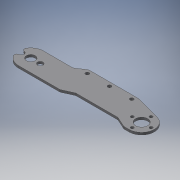
# Autodesk Inventor part: rinnku
Saved by Autodesk Inventor 2018 (Build 220112000, 112)
## iProperties
Created: 2016-08-23
Part Number: rinnku
Material: GFRP
Document SubType Name: Modeling
Designer: hiro
Density: 1.75 g/cm^3
Appearance: 滑らか - 淡い灰色
Mass: 9.22094 g
Surface Area: 59.6576 cm^2
Volume: 5.26911 cm^3
Author: hiro
Autodesk Inventor part; units mm, degrees
ref_plane "YZ Plane" through (0, 0, 0) normal (1, 0, 0) x (0, 1, 0)
ref_plane "XZ Plane" through (0, 0, 0) normal (0, 1, 0) x (-1, 0, 0)
ref_plane "XY Plane" through (0, 0, 0) normal (0, 0, 1) x (1, 0, 0)
sketch "スケッチ1" plane through (0, 0, 0) normal (0, 0, 1) x (1, 0, 0)
  line L0 (-50, 0) -> (50, 0) construction
  circle A0 centre (-50, 0) radius 4
  circle A1 centre (50, 0) radius 5.55
  line L1 (-50, 11.35) -> (-23, 11.35)
  line L2 (-50, -11.35) -> (50, -11.35)
  arc A2 (50, -11.35) -> (50, 11.35) centre (50, 0) ccw
  line L3 (30, 17) -> (-15, 17)
  line L4 (-15, 17) -> (-23, 11.35)
  line L5 (-24.9115, 10) -> (41.8474, 10) construction
  line L6 (-15, 17) -> (-15, 10) construction
  line L7 (30, 17) -> (30, 10) construction
  circle A3 centre (27.5, 13.5) radius 1.55
  circle A4 centre (-12.5, 13.5) radius 1.55
  circle A5 centre (7.5, 13.5) radius 1.55
  line L8 (-15, 13.5) -> (30, 13.5) construction
  line L9 (30, 16) -> (-15, 16) construction
  line L10 (-15, 16) -> (-15, 11) construction
  line L11 (-15, 11) -> (30, 11) construction
  line L12 (30, 11) -> (30, 16) construction
  line L13 (-23, 11.35) -> (50, 11.35)
  arc A6 (-50, 11.35) -> (-50, -11.35) centre (-50, 0) ccw
  line L14 (7.5, 17) -> (7.5, 10.5172) construction
  line L15 (30, 17) -> (52.8887, 10.9762)
  point P0 (0, 0)
  point P1 (0, 0)
  point P2 (55.7736, 9.7718)
  point P3 (38, 11.35)
  dimension "d0" = 100
  dimension "d1" = 8
  dimension "d8" = 11.1
  dimension "d10" = 7
  dimension "d11" = 45
  dimension "d12" = 2.5
  dimension "d13" = 3.1
  dimension "d14" = 2.5
  dimension "d15" = 20
  dimension "d17" = 5
  dimension "d18" = 11
  dimension "d69" = 11.35
  dimension "d72" = 11.35
  dimension "d87" = 8
  dimension "d88" = 8
  constraints: 32 end point, 8 point on line, 7 centre point, 7 horizontal, 6 midpoint, 6 point on circle, 5 coincident, 4 perpendicular, 4 tangent, 2 equal radius, 2 parallel
  measures "d0" distance of L0.start L0.end
  measures "d1" diameter of A0
  measures "d8" diameter of A1
  measures "d10" distance between parallel lines of L3 L5
  measures "d11" distance between parallel lines of L7 L6
  measures "d12" distance from line of A4.centre L6
  measures "d13" diameter of A4
  measures "d14" distance from line of L7 A3.centre
  measures "d15" distance from line of L7 L0.end
  measures "d17" distance between parallel lines of L9 L11
  measures "d18" distance between parallel lines of L0 L11
  measures "d69" radius of A2
  measures "d72" radius of A6
  measures "d87" horizontal distance of L3.start point (38, 11.35)
  measures "d88" horizontal distance of L3.end L1.end
extrude "押し出し1" add sketch "スケッチ1" along normal blind 2
fillet "フィレット1" radius 5 3 edges at (-23, 11.35, 1) (-15, 17, 1) (30, 17, 1)
sketch "スケッチ2" plane through (0, 0, 2) normal (0, 0, 1) x (1, 0, 0)
  arc A0 (50, -11.35) -> (52.8887, 10.9762) centre (50, 0) ccw projected
  line L0 (18, -20) -> (-35.4549, -20) construction
  line L1 (-76.9372, -11.5) -> (-72, -11.5)
  line L2 (-76.9372, -12.4) -> (-76.9372, -11.5)
  line L3 (-71.9872, -11.45) -> (-76.9872, -11.45)
  line L4 (-76.9872, -11.45) -> (-76.9872, -12.45)
  circle A1 centre (-50, 0) radius 4 projected
  circle A2 centre (-50, 0) radius 5.5 construction
  circle A3 centre (50, 0) radius 5.55 projected
  line L5 (83.3205, -17.7128) -> (50, 0) construction
  line L6 (50, 0) -> (18, -20) construction
  line L7 (83.3205, -17.7128) -> (37.8533, -17.7128) construction
  line L8 (-13.4166, -12.4128) -> (46.4577, -12.4128)
  line L9 (46.4577, -12.4128) -> (46.4577, -11.5128)
  line L10 (46.4577, -11.5128) -> (45.5205, -11.5128)
  line L11 (45.5205, -11.5128) -> (35.5205, -7.0128)
  line L12 (35.5205, -7.0128) -> (-2.4795, -7.0128)
  line L13 (-2.4795, -7.0128) -> (-12.4795, -11.5128)
  line L14 (-12.4795, -11.5128) -> (-13.4166, -11.5128)
  line L15 (-13.4166, -11.5128) -> (-13.4166, -12.4128)
  line L16 (-12.4902, -11.4628) -> (-2.4902, -6.9628)
  line L17 (-2.4902, -6.9628) -> (35.5312, -6.9628)
  line L18 (35.5312, -6.9628) -> (45.5312, -11.4628)
  line L19 (45.5312, -11.4628) -> (46.5077, -11.4628)
  line L20 (46.5077, -11.4628) -> (46.5077, -12.4628)
  line L21 (46.5077, -12.4628) -> (-13.4666, -12.4628)
  line L22 (-13.4666, -12.4628) -> (-13.4666, -11.4628)
  line L23 (-13.4666, -11.4628) -> (-12.4902, -11.4628)
  point P0 (56.6914, 9.1677)
  point P1 (0, 0)
  point P2 (50, 11.35)
  dimension "d19" = 20
  dimension "d20" = 32
  dimension "d32" = 11
  dimension "d33" = 120
  dimension "d37" = 37.8
  dimension "d38" = 6.2
  dimension "d39" = 0.05
  dimension "d49" = 38
  dimension "d50" = 10
  dimension "d51" = 10
  dimension "d52" = 4.5
  dimension "d53" = 0.9
  dimension "d54" = 59.9743
  constraints: 48 end point, 6 horizontal, 4 perpendicular, 3 equal length, 2 collinear, 1 centre point, 1 coincident, 1 horizontal alignment, 8 other
  measures "d19" vertical distance of A0.centre L0.start
  measures "d20" horizontal distance of L0.start A0.centre
  measures "d32" diameter of A2
  measures "d33" angle of L6 L5
  measures "d37" horizontal distance of L5.start L10.end
  measures "d38" distance from line of L10 L5.start
  measures "d39" distance between parallel lines of L16 L13
  measures "d49" distance of L11.end L12.end
  measures "d50" horizontal distance of L12.end L13.end
  measures "d51" horizontal distance of L10.end L11.end
  measures "d52" distance from line of L10.end L12
  measures "d53" distance between parallel lines of L8 L10
  measures "d54" distance between parallel lines of L22 L20
extrude "押し出し2" cut sketch "スケッチ2" against normal blind 10 contours L15 L14 L13 L12 L11 L10 L9 L8 | L16 L17 L18 L19 L20 L21 L22 L23
fillet "フィレット2" radius 2 4 edges at (-12.2395, -11.35, 1) (-2.4902, -6.9628, 1) (45.2805, -11.35, 1) (35.5312, -6.9628, 1)
sketch "スケッチ4" plane through (0, 0, 2) normal (0, 0, 1) x (1, 0, 0)
  circle A0 centre (50, 0) radius 5.55 projected
  circle A1 centre (50, 0) radius 8.5 construction
  line L0 (50, 0) -> (50, 8.5) construction
  circle A2 centre (50, 8.5) radius 1.35
  circle A3 centre (41.5, 0) radius 1.35
  circle A4 centre (50, -8.5) radius 1.35
  circle A5 centre (58.5, 0) radius 1.35
  point P0 (0, 0)
  dimension "d61" = 17
  dimension "d62" = 2.7
  dimension "d65" = 360
  constraints: 4 centre point, 2 coincident, 2 end point, 1 vertical, 1 vertical alignment, 11 other
  measures "d62" diameter of A2
extrude "押し出し4" cut sketch "スケッチ4" against normal through all contours A2 | A3 | A4 | A5
sketch "スケッチ6" plane through (0, 0, 2) normal (0, 0, 1) x (1, 0, 0)
  circle A0 centre (-50, 0) radius 4 projected
  circle A1 centre (-50, 0) radius 8.5 construction
  circle A2 centre (-58.5, 0) radius 2.5
  line L0 (-50, 0) -> (-58.5, 0) construction
  line L1 (-50, 0) -> (-41.5, 0) construction
  circle A3 centre (-41.5, 0) radius 2.5
  arc A4 (-50, 11.35) -> (-50, -11.35) centre (-50, 0) ccw projected
  line L2 (-58.5, -2.5) -> (-61.0712, -2.5)
  line L3 (-58.5, 2.5) -> (-61.0712, 2.5)
  point P0 (0, 0)
  dimension "d78" = 17
  dimension "d79" = 5
  dimension "d82" = 360
  constraints: 8 end point, 4 point on circle, 2 centre point, 2 horizontal, 2 tangent, 1 coincident, 1 horizontal alignment, 12 other
  measures "d79" diameter of A2
extrude "押し出し6" cut sketch "スケッチ6" against normal through all contours A2 | A2 L2 A4 L3 | A3
fillet "フィレット4" radius 2 2 edges at (-61.0712, 2.5, 1) (-61.0712, -2.5, 1)
equation "\"d14\" = d12"
